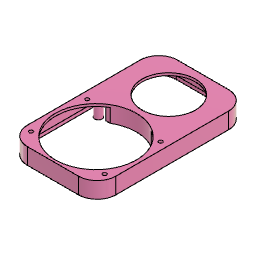
Gehaeuse_oben (Autodesk Fusion 360 design; units mm, degrees)
Autodesk Fusion 360 part; units mm, degrees
sketch "Skizze1" plane through (0, 0, 0) normal (0, 0, 1) x (1, 0, 0)
  circle A0 centre (0, 0) radius 32.5
  line L0 (20.5, -34.5) -> (-20.5, -34.5)
  line L1 (-35.5, -19.5) -> (-35.5, 71)
  line L2 (-20.5, 86) -> (20.5, 86)
  line L3 (35.5, 71) -> (35.5, -19.5)
  line L4 (35.5, -34.5) -> (-35.5, 86) construction
  line L5 (-35.5, -34.5) -> (35.5, 86) construction
  circle A1 centre (0, 58.5) radius 21.5
  arc A2 (20.5, -34.5) -> (35.5, -19.5) centre (20.5, -19.5) ccw
  arc A3 (-35.5, -19.5) -> (-20.5, -34.5) centre (-20.5, -19.5) ccw
  arc A4 (-20.5, 86) -> (-35.5, 71) centre (-20.5, 71) ccw
  arc A5 (35.5, 71) -> (20.5, 86) centre (20.5, 71) ccw
  point P0 (0, 25.75)
  dimension "d1" = 65
  dimension "d2" = 71
  dimension "d3" = 120.5
  dimension "d4" = 34.5
  dimension "d5" = 43
  dimension "d6" = 27.5
  dimension "d7" = 15
  dimension "d8" = 15
  dimension "d9" = 15
  dimension "d10" = 15
  constraint coincident A0.centre origin
  constraint horizontal L0
  constraint perpendicular L0 L1
  constraint parallel L0 L2
  constraint parallel L1 L3
  constraint coincident L4 P0
  constraint coincident L5 P0
  constraint vertical A0.centre P0
  constraint vertical A0.centre A1.centre
  constraint coincident L4.start L0
  constraint coincident L4.start L3
  constraint tangent L0 A2
  constraint tangent L3 A2
  constraint coincident L5.start L1
  constraint coincident L5.start L0
  constraint tangent L1 A3
  constraint tangent L0 A3
  constraint coincident L4.end L1
  constraint coincident L4.end L2
  constraint tangent L1 A4
  constraint tangent L2 A4
  constraint coincident L5.end L2
  constraint coincident L5.end L3
  constraint tangent L2 A5
  constraint tangent L3 A5
  measures "d1" diameter of A0
  measures "d2" distance of L4.start L5.start
  measures "d3" distance of L4.start L5.end
  measures "d4" distance of A0.centre L0
  measures "d5" diameter of A1
  measures "d6" distance of L2 A1.centre
  measures "d7" radius of A2
  measures "d8" radius of A3
  measures "d9" radius of A4
  measures "d10" radius of A5
extrude "Extrusion1" add sketch "Skizze1" against normal blind 13
shell "Schale1" thickness 2 removed faces 1 at (-27.6325, 47.1569, -13)
sketch "Skizze2" plane through (0, 0, -13) normal (0, 0, -1) x (1, 0, 0)
  line L0 (11.5758, 32.5) -> (20.5, 32.5)
  arc A0 (33.5, 19.5) -> (20.5, 32.5) centre (20.5, 19.5) ccw
  line L1 (33.5, 19.5) -> (33.5, 8.2462)
  arc A1 (33.5, 8.2462) -> (11.5758, 32.5) centre (0, 0) ccw
  arc A2 (35.5, 19.5) -> (20.5, 34.5) centre (20.5, 19.5) ccw
  line L2 (20.5, 34.5) -> (-20.5, 34.5)
  arc A3 (-20.5, 34.5) -> (-35.5, 19.5) centre (-20.5, 19.5) ccw
  line L3 (-35.5, 19.5) -> (-35.5, -71)
  arc A4 (-35.5, -71) -> (-20.5, -86) centre (-20.5, -71) ccw
  line L4 (-20.5, -86) -> (20.5, -86)
  arc A5 (20.5, -86) -> (35.5, -71) centre (20.5, -71) ccw
  line L5 (35.5, -71) -> (35.5, 19.5)
  circle A6 centre (0, 0) radius 32.5
  line L6 (-33.5, 8.2462) -> (-33.5, 19.5)
  arc A7 (-20.5, 32.5) -> (-33.5, 19.5) centre (-20.5, 19.5) ccw
  line L7 (-20.5, 32.5) -> (-11.5758, 32.5)
  arc A8 (-11.5758, 32.5) -> (-33.5, 8.2462) centre (0, 0) ccw
  line L8 (20.5, -84) -> (-20.5, -84)
  arc A9 (-33.5, -71) -> (-20.5, -84) centre (-20.5, -71) ccw
  line L9 (-33.5, -71) -> (-33.5, -8.2462)
  arc A10 (-33.5, -8.2462) -> (33.5, -8.2462) centre (0, 0) ccw
  line L10 (33.5, -8.2462) -> (33.5, -71)
  arc A11 (20.5, -84) -> (33.5, -71) centre (20.5, -71) ccw
  circle A12 centre (0, -58.5) radius 23.5
  circle A13 centre (0, -58.5) radius 21.5
  line L11 (-33.5, 8.2462) -> (-33.5, -8.2462)
  line L12 (33.5, 8.2462) -> (33.5, -8.2462)
  line L13 (-11.5758, 32.5) -> (11.5758, 32.5)
  line L14 (-20.1556, -28) -> (20.1556, -28)
  dimension "d14" = 58
  constraint coincident L6.start A8.end
  constraint coincident L9.end A10.start
  constraint coincident L1.end A1.start
  constraint coincident A10.end L10.start
  constraint coincident L7.end A8.start
  constraint coincident L0.start A1.end
  constraint coincident A10 L14.start
  constraint coincident A10 L14.end
  constraint horizontal L14
  measures "d14" distance of L4 L14
extrude "Extrusion2" cut sketch "Skizze2" against normal up to surface (11 mm away) contours A1 A6 A10 L12 L13 L14 | A6 A8 A10 L11 L13 L14 | A12
sketch "Skizze3" plane through (0, 0, -13) normal (0, 0, -1) x (1, 0, 0)
  arc A0 (35.5, 19.5) -> (20.5, 34.5) centre (20.5, 19.5) ccw
  line L0 (20.5, 34.5) -> (-20.5, 34.5)
  arc A1 (-20.5, 34.5) -> (-35.5, 19.5) centre (-20.5, 19.5) ccw
  line L1 (-35.5, 19.5) -> (-35.5, -71)
  arc A2 (-35.5, -71) -> (-20.5, -86) centre (-20.5, -71) ccw
  line L2 (-20.5, -86) -> (20.5, -86)
  arc A3 (20.5, -86) -> (35.5, -71) centre (20.5, -71) ccw
  line L3 (35.5, -71) -> (35.5, 19.5)
  line L4 (-33.5, -71) -> (-33.5, 19.5)
  arc A4 (-20.5, 32.5) -> (-33.5, 19.5) centre (-20.5, 19.5) ccw
  line L5 (-20.5, 32.5) -> (20.5, 32.5)
  arc A5 (33.5, 19.5) -> (20.5, 32.5) centre (20.5, 19.5) ccw
  line L6 (33.5, 19.5) -> (33.5, -71)
  arc A6 (20.5, -84) -> (33.5, -71) centre (20.5, -71) ccw
  line L7 (20.5, -84) -> (-20.5, -84)
  arc A7 (-33.5, -71) -> (-20.5, -84) centre (-20.5, -71) ccw
  arc A8 (-20.5, 33.5) -> (-34.5, 19.5) centre (-20.5, 19.5) ccw
  line L8 (-34.5, -71) -> (-34.5, 19.5)
  arc A9 (-34.5, -71) -> (-20.5, -85) centre (-20.5, -71) ccw
  line L9 (20.5, -85) -> (-20.5, -85)
  arc A10 (20.5, -85) -> (34.5, -71) centre (20.5, -71) ccw
  line L10 (34.5, 19.5) -> (34.5, -71)
  arc A11 (34.5, 19.5) -> (20.5, 33.5) centre (20.5, 19.5) ccw
  line L11 (-20.5, 33.5) -> (20.5, 33.5)
  dimension "d17" = -1
extrude "Extrusion3" cut sketch "Skizze3" against normal blind 3.75 contours A8 L8 A9 L9 A10 L10 A11 L11
sketch "Skizze4" plane through (0, 0, -2) normal (0, 0, -1) x (1, 0, 0)
  circle A0 centre (0, -58.5) radius 21.5
  line L0 (-33.5, 19.5) -> (-33.5, -71)
  arc A1 (-33.5, -71) -> (-20.5, -84) centre (-20.5, -71) ccw
  line L1 (-20.5, -84) -> (20.5, -84)
  arc A2 (20.5, -84) -> (33.5, -71) centre (20.5, -71) ccw
  line L2 (33.5, -71) -> (33.5, 19.5)
  arc A3 (33.5, 19.5) -> (20.5, 32.5) centre (20.5, 19.5) ccw
  line L3 (20.5, 32.5) -> (0, 32.5)
  arc A4 (16.5, -28) -> (0, 32.5) centre (0, 0) ccw
  line L4 (16.5, -28) -> (20.1556, -28)
  arc A5 (-20.1556, -28) -> (20.1556, -28) centre (0, 0) ccw
  line L5 (-20.1556, -28) -> (-16.5, -28)
  arc A6 (0, 32.5) -> (-16.5, -28) centre (0, 0) ccw
  line L6 (0, 32.5) -> (-20.5, 32.5)
  arc A7 (-20.5, 32.5) -> (-33.5, 19.5) centre (-20.5, 19.5) ccw
  circle A8 centre (-26.5, -28.5) radius 3
  circle A9 centre (-26.5, -28.5) radius 1.15
  line L7 (-35.5, 19.5) -> (-35.5, -71)
  circle A10 centre (26.5, -28.5) radius 3
  circle A11 centre (26.5, -28.5) radius 1.15
  line L8 (35.5, -71) -> (35.5, 19.5)
  line L9 (-20.5, -86) -> (20.5, -86)
  dimension "d20" = 6
  dimension "d21" = 2.3
  dimension "d22" = 9
  dimension "d23" = 9
  dimension "d24" = 57.5
  constraint concentric A8 A9
  constraint concentric A10 A11
  constraint equal A8 A10
  constraint equal A9 A11
  constraint horizontal A8.centre A10.centre
  measures "d20" diameter of A8
  measures "d21" diameter of A9
  measures "d22" distance of A8.centre L7
  measures "d23" distance of A10.centre L8
  measures "d24" distance of A8.centre L9
extrude "Extrusion4" add sketch "Skizze4" along normal blind 11.75 contours A8 | A10
sketch "Skizze5" plane through (0, 0, 0) normal (0, 0, 1) x (1, 0, 0)
  circle A0 centre (-26.5, 28.5) radius 3
  circle A1 centre (0, 58.5) radius 21.5
  line L0 (-33.5, -19.5) -> (-33.5, 71)
  arc A2 (-20.5, 84) -> (-33.5, 71) centre (-20.5, 71) ccw
  line L1 (-20.5, 84) -> (20.5, 84)
  arc A3 (33.5, 71) -> (20.5, 84) centre (20.5, 71) ccw
  line L2 (33.5, 71) -> (33.5, -19.5)
  arc A4 (20.5, -32.5) -> (33.5, -19.5) centre (20.5, -19.5) ccw
  line L3 (20.5, -32.5) -> (0, -32.5)
  arc A5 (0, -32.5) -> (16.5, 28) centre (0, 0) ccw
  line L4 (16.5, 28) -> (20.1556, 28)
  arc A6 (20.1556, 28) -> (-20.1556, 28) centre (0, 0) ccw
  line L5 (-20.1556, 28) -> (-16.5, 28)
  arc A7 (-16.5, 28) -> (0, -32.5) centre (0, 0) ccw
  line L6 (0, -32.5) -> (-20.5, -32.5)
  arc A8 (-33.5, -19.5) -> (-20.5, -32.5) centre (-20.5, -19.5) ccw
  circle A9 centre (26.5, 28.5) radius 3
  line L7 (0, -31.5) -> (-20.5, -31.5)
  arc A10 (-32.5, -19.5) -> (-20.5, -31.5) centre (-20.5, -19.5) ccw
  line L8 (-32.5, -19.5) -> (-32.5, 24.5)
  line L9 (32.5, 24.5) -> (32.5, -19.5)
  arc A11 (20.5, -31.5) -> (32.5, -19.5) centre (20.5, -19.5) ccw
  line L10 (20.5, -31.5) -> (0, -31.5)
  line L11 (-19.799, 24.5) -> (-32.5, 24.5)
  line L12 (19.799, 24.5) -> (32.5, 24.5)
  arc A12 (19.799, 24.5) -> (-19.799, 24.5) centre (0, 0) ccw
  point P0 (-32.5, -31.5)
  dimension "d57" = 63
  dimension "d58" = 1
  dimension "d59" = 4
  constraint concentric A5 A12
  constraint perpendicular L8 L11
  constraint perpendicular L9 L12
  constraint parallel L6 L7
  constraint concentric A8 A10
  constraint parallel L0 L8
  constraint parallel L2 L9
  constraint concentric A4 A11
  constraint parallel L3 L10
  constraint tangent A10 L8
  constraint tangent L7 A10
  constraint tangent L9 A11
  constraint tangent A11 L10
  constraint horizontal L11.start L12.start
  constraint vertical A10.start P0
  constraint horizontal L7.end P0
  measures "d57" diameter of A12
  measures "d58" distance of L0 L8
  measures "d59" distance of A0.centre L11
sketch "Skizze6" plane through (0, 0, 0) normal (0, 0, 1) x (-1, 0, 0)
  circle A0 centre (0, 0) radius 32.5
  circle A1 centre (0, -58.5) radius 21.5
  arc A2 (-20.5, 34.5) -> (-35.5, 19.5) centre (-20.5, 19.5) ccw
  line L0 (-35.5, 19.5) -> (-35.5, -71)
  arc A3 (-35.5, -71) -> (-20.5, -86) centre (-20.5, -71) ccw
  line L1 (-20.5, -86) -> (20.5, -86)
  arc A4 (20.5, -86) -> (35.5, -71) centre (20.5, -71) ccw
  line L2 (35.5, -71) -> (35.5, 19.5)
  arc A5 (35.5, 19.5) -> (20.5, 34.5) centre (20.5, 19.5) ccw
  line L3 (20.5, 34.5) -> (-20.5, 34.5)
  circle A6 centre (0, 0) radius 30.5
  line L4 (-6.16, 14.63) -> (-6.16, -29.8715)
  line L5 (-4.16, 12.63) -> (-4.16, -14.67)
  line L6 (-6.16, 14.63) -> (26.7622, 14.63)
  line L7 (28.14, 12.63) -> (-4.16, 12.63)
  point P0 (32.5, 31.5)
  dimension "d60" = -2
  dimension "d61" = 2
  dimension "d62" = 2
  constraint coincident A6 L4.end
  constraint vertical L4
  constraint coincident A6 L6.end
  constraint perpendicular L4 L6
  measures "d61" distance of L4 L5
  measures "d62" distance of L6 L7
sketch "Skizze7" plane through (0, 0, 0) normal (0, 0, 1) x (-1, 0, 0)
  circle A0 centre (0, 0) radius 32.5
  circle A1 centre (0, -58.5) radius 21.5
  arc A2 (-20.5, 34.5) -> (-35.5, 19.5) centre (-20.5, 19.5) ccw
  line L0 (-35.5, 19.5) -> (-35.5, -71)
  arc A3 (-35.5, -71) -> (-20.5, -86) centre (-20.5, -71) ccw
  line L1 (-20.5, -86) -> (20.5, -86)
  arc A4 (20.5, -86) -> (35.5, -71) centre (20.5, -71) ccw
  line L2 (35.5, -71) -> (35.5, 19.5)
  arc A5 (35.5, 19.5) -> (20.5, 34.5) centre (20.5, 19.5) ccw
  line L3 (20.5, 34.5) -> (-20.5, 34.5)
  circle A6 centre (29.5, 22.5) radius 1.25
  circle A7 centre (29.5, -22.5) radius 1.25
  circle A8 centre (-29.5, -22.5) radius 1.25
  circle A9 centre (-29.5, 22.5) radius 1.25
  circle A10 centre (29.5, -22.5) radius 1.5
  circle A11 centre (-29.5, -22.5) radius 1.5
  circle A12 centre (-29.5, 22.5) radius 1.5
  circle A13 centre (29.5, 22.5) radius 1.5
  dimension "d177" = 3
  dimension "d178" = 3
  dimension "d179" = 3
  dimension "d180" = 3
  constraint concentric A7 A10
  constraint concentric A8 A11
  constraint concentric A9 A12
  constraint concentric A6 A13
  measures "d177" diameter of A10
  measures "d178" diameter of A11
  measures "d179" diameter of A13
  measures "d180" diameter of A12
extrude "Extrusion5" cut sketch "Skizze7" against normal up to surface (2 mm away) contours A6 | A7 | A8 | A9 | A10 | A11 | A12 | A13
equation "d4 = ( d1 / 2 ) + 2 mm"
equation "d6 = ( d5 / 2 ) + 6 mm"
equation "d8 = d7"
equation "d9 = d7"
equation "d10 = d7"
equation "d22 = 12 mm - ( d20 / 2 )"
equation "d23 = d22"
equation "d24 = 60.5 mm - ( d20 / 2 )"
equation "d62 = d61"
equation "d178 = d177"
equation "d179 = d177"
equation "d180 = d177"
